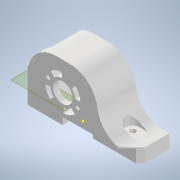
# Autodesk Inventor part: Intake90tdriev
Saved by Autodesk Inventor 2020 (Build 240168000, 168)
## iProperties
Created: 2020-03-03
Part Number: Intake90tdriev
Material: Generic
Document SubType Name: Modeling
Designer: srini
Density: 1 g/cm^3
Appearance: Default
Author: srini
Autodesk Inventor part; units mm, degrees
ref_plane "YZ Plane" through (0, 0, 0) normal (1, 0, 0) x (0, 1, 0)
ref_plane "XZ Plane" through (0, 0, 0) normal (0, 1, 0) x (-1, 0, 0)
ref_plane "XY Plane" through (0, 0, 0) normal (0, 0, 1) x (1, 0, 0)
sketch "Sketch1" plane through (0, 0, 0) normal (0, 0, 1) x (1, 0, 0)
  circle A0 centre (-31.75, -41.275) radius 14.2875 projected
  circle A1 centre (-18.8128, 31.24) radius 8.75 construction
  circle A2 centre (-18.8128, 31.24) radius 8.95
  line L0 (-50.5628, 57.15) -> (12.9372, 57.15)
  line L1 (12.9372, 57.15) -> (12.9372, 0)
  line L2 (12.9372, 0) -> (-50.5628, 0)
  line L3 (-50.5628, 0) -> (-50.5628, 57.15)
  line L4 (450.85, 0) -> (-107.95, 0) projected
  circle A3 centre (-18.8128, 31.24) radius 22.15 construction
  circle A4 centre (-18.8128, 31.24) radius 22.35
  line L5 (-50.5628, 0) -> (-63.5, 0)
  line L6 (-63.5, 0) -> (-63.5, 25.4)
  line L7 (-63.5, 25.4) -> (-50.5628, 25.4)
  line L8 (-50.5628, 25.4) -> (-50.5628, 0)
  line L9 (12.9372, 0) -> (43.4172, 0)
  line L10 (43.4172, 0) -> (43.4172, 12.7)
  line L11 (43.4172, 12.7) -> (12.9372, 12.7)
  line L12 (12.9372, 12.7) -> (12.9372, 0)
  line L13 (-63.5, -1.5266) -> (-63.5, -23.8734) projected
  point P0 (0, 0)
  point P1 (-50.5628, 25.4)
  point P2 (-50.5628, 0)
  point P3 (12.9372, 0)
  point P4 (43.4172, 0)
  point P5 (12.9372, 12.7)
  dimension "d0" = 17.5
  dimension "d1" = 17.9
  dimension "d2" = 73.66
  dimension "d3" = 57.15
  dimension "d4" = 44.3
  dimension "d5" = 44.7
  dimension "d6" = 63.5
  dimension "d7" = 31.75
  dimension "d8" = 25.4
  dimension "d58" = 12.7
  dimension "d59" = 30.48
  dimension "d71" = 31.24
  constraints: 24 end point, 6 parallel, 3 horizontal, 3 perpendicular, 2 centre point, 2 collinear, 1 coincident
  measures "d0" diameter of A1
  measures "d1" diameter of A2
  measures "d2" distance of A0.centre A2.centre
  measures "d3" distance of L2.end L0.start
  measures "d4" diameter of A3
  measures "d5" diameter of A4
  measures "d6" distance of L0.start L0.end
  measures "d7" distance from line of A2.centre L3
  measures "d8" distance of L5.end L6.end
  measures "d58" distance of L9.end L10.end
  measures "d59" distance of L10.end L11.end
  measures "d71" vertical distance of point (0, 0) A4.centre
extrude "Extrusion1" add sketch "Sketch1" against normal blind 25.4 contours L0 L1 L2 L3 | L3 L4 L6 L7 | L11 L10 L4 L1 | A4
sketch "Sketch2" plane through (0, 0, -25.4) normal (0, 0, -1) x (-1, 0, 0)
  circle A0 centre (18.8128, 31.24) radius 8.95 projected
  circle A1 centre (18.8128, 31.24) radius 22.35
  point P0 (0, 0)
  dimension "d12" = 44.7
  constraints: 1 centre point, 1 coincident
  measures "d12" diameter of A1
extrude "Extrusion2" cut sketch "Sketch2" against normal blind 20.32
sketch "Sketch3" plane through (0, 0, -25.4) normal (0, 0, -1) x (-1, 0, 0)
  line L0 (-43.4172, 0) -> (63.5, 0) projected
  circle A0 centre (18.8128, 31.24) radius 22.35 projected
  line L1 (63.5, 0) -> (63.5, 25.4) projected
  line L2 (63.5, 25.4) -> (50.5628, 25.4) projected
  line L3 (50.5628, 25.4) -> (50.5628, 57.15) projected
  line L4 (50.5628, 57.15) -> (-12.9372, 57.15) projected
  line L5 (-12.9372, 57.15) -> (-12.9372, 12.7) projected
  line L6 (-12.9372, 12.7) -> (-43.4172, 12.7) projected
  line L7 (-43.4172, 12.7) -> (-43.4172, 0) projected
  point P0 (0, 0)
ref_plane "Work Plane1" through (-63.5004, -61.913, -35.052) normal (0, 0, -1) x (0, 1, 0)
extrude "Extrusion3" add sketch "Sketch3" along normal up to surface (9.652 mm away)
fillet "Fillet1" radius 25.4 2 edges at (-50.5628, 57.15, -17.526) (12.9372, 57.15, -17.526)
fillet "Fillet2" radius 25.4 2 edges at (-50.5628, 25.4, -17.526) (12.9372, 12.7, -17.526)
chamfer "Chamfer1" distance 12.7 angle 45 2 edges at (-63.5, 12.7, 0) (43.4172, 6.35, 0)
sketch "Sketch4" plane through (-63.5, 25.4, -35.052) normal (0, 1, 0) x (1, 0, 0)
  line L0 (514.35, -2.286) -> (-44.45, -2.286) projected
  line L1 (0, -22.352) -> (0, 0) projected
  line L2 (116.9864, -22.352) -> (116.9864, 0) projected
  circle A0 centre (12.2114, -14.986) radius 2.5781
  circle A1 centre (102.3814, -14.986) radius 2.5781
  line L3 (63.7064, -35.052) -> (45.8064, -35.052) projected
  line L4 (54.7564, -35.052) -> (54.7564, -21.2644)
  point P0 (63.5, -35.052)
  dimension "d26" = 42.545
  dimension "d27" = 47.625
  dimension "d28" = 12.7
  dimension "d29" = 12.7
  dimension "d30" = 5.1562
  constraints: 2 centre point, 2 end point, 1 equal radius, 1 midpoint, 1 vertical
  measures "d26" distance from line of A0.centre L4
  measures "d27" distance from line of A1.centre L4
  measures "d28" distance from line of A0.centre L0
  measures "d29" distance from line of A1.centre L0
  measures "d30" diameter of A0
extrude "Extrusion4" [suppressed]
sketch "Sketch5" plane through (-63.5, 25.4, -35.052) normal (0, 1, 0) x (1, 0, 0)
  circle A0 centre (12.2114, -14.986) radius 2.5781 projected
  circle A1 centre (12.2114, -14.986) radius 6.35
  circle A2 centre (102.3814, -14.986) radius 2.5781 projected
  circle A3 centre (102.3814, -14.986) radius 6.35
  point P0 (63.5, -35.052)
  point P1 (0, -15.9438)
  point P2 (0, -14.0282)
  dimension "d33" = 12.7
  dimension "d34" = 12.7
  constraints: 2 centre point, 2 coincident, 1 other
  measures "d33" diameter of A1
  measures "d34" diameter of A3
extrude "Extrusion5" [suppressed]
sketch "Sketch6" plane through (0, 0, 0) normal (0, 0, 1) x (1, 0, 0)
  line L0 (-17.8812, 15.2671) -> (-18.1549, 19.9592) projected
  arc A0 (-17.8812, 15.2671) -> (-7.832, 19.6029) centre (-18.8128, 31.24) ccw projected
  line L1 (-7.832, 19.6029) -> (-11.0576, 23.0213) projected
  arc A1 (-18.1549, 19.9592) -> (-11.0576, 23.0213) centre (-18.8128, 31.24) ccw projected
  line L2 (-2.84, 32.1716) -> (-7.532, 31.898) projected
  arc A2 (-2.84, 32.1716) -> (-7.1758, 42.2208) centre (-18.8128, 31.24) ccw projected
  line L3 (-7.1758, 42.2208) -> (-10.5941, 38.9952) projected
  arc A3 (-7.532, 31.898) -> (-10.5941, 38.9952) centre (-18.8128, 31.24) ccw projected
  line L4 (-19.4708, 42.5208) -> (-19.7445, 47.2129) projected
  arc A4 (-19.7445, 47.2129) -> (-29.7937, 42.8771) centre (-18.8128, 31.24) ccw projected
  line L5 (-26.568, 39.4587) -> (-29.7937, 42.8771) projected
  arc A5 (-19.4708, 42.5208) -> (-26.568, 39.4587) centre (-18.8128, 31.24) ccw projected
  line L6 (-30.0937, 30.582) -> (-34.7857, 30.3084) projected
  arc A6 (-34.7857, 30.3084) -> (-30.4499, 20.2592) centre (-18.8128, 31.24) ccw projected
  line L7 (-27.0315, 23.4848) -> (-30.4499, 20.2592) projected
  arc A7 (-30.0937, 30.582) -> (-27.0315, 23.4848) centre (-18.8128, 31.24) ccw projected
  circle A8 centre (-32.2888, 36.5924) radius 1.65 projected
  circle A9 centre (-5.3368, 25.8876) radius 1.65 projected
  point P0 (0, 0)
extrude "Extrusion6" cut sketch "Sketch6" against normal through all
sketch "Sketch7" plane through (43.4172, 0, -35.052) normal (0, 0, -1) x (-1, 0, 0)
  line L0 (92.2212, 54.3381) -> (76.8128, 48.2059)
  line L1 (76.8128, 48.2059) -> (84.487, 28.923)
  line L2 (84.487, 28.923) -> (99.8954, 35.0553)
  line L3 (99.8954, 35.0553) -> (92.2212, 54.3381)
  line L4 (86.8955, 49.4848) -> (86.916, 49.5323) projected
  line L5 (86.8955, 49.4848) -> (83.8448, 48.2707) projected
  line L6 (83.8448, 48.2707) -> (83.7035, 48.2517) projected
  line L7 (83.7035, 48.2517) -> (80.1568, 46.8402) projected
  line L8 (80.1542, 46.8413) -> (80.1568, 46.8402) projected
  line L9 (80.1542, 46.8413) -> (86.916, 49.5323) projected
  line L10 (92.7253, 34.9354) -> (92.6777, 34.9559) projected
  line L11 (92.7253, 34.9354) -> (85.9635, 32.2444) projected
  line L12 (85.9635, 32.2444) -> (85.9646, 32.247) projected
  line L13 (85.9646, 32.247) -> (89.5113, 33.6585) projected
  line L14 (89.5113, 33.6585) -> (89.627, 33.7418) projected
  line L15 (89.627, 33.7418) -> (92.6777, 34.9559) projected
  point P0 (43.4172, 0)
  dimension "d39" = 2.54
  dimension "d40" = 2.54
  constraints: 8 end point, 3 parallel, 1 perpendicular
  measures "d39" distance between parallel lines of L0 L5
  measures "d40" distance between parallel lines of L2 L11
extrude "Extrusion7" cut sketch "Sketch7" against normal blind 25.4 contours L3 L2 L1 L0 | L5 L6 L9 L4 | L11 L12 L13 L14 L15 L10
fillet "Fillet3" radius 6.35 2 edges at (-33.4044, 48.1839, -9.652) (-41.059, 28.9504, -9.652)
fillet "Fillet4" radius 2.54 1 edges at (-41.311, 51.356, -22.352)
fillet "Fillet5" radius 2.54 2 edges at (-37.5848, 53.9052, -9.6617) (-44.724, 47.9525, -9.652)
sketch "Sketch8" plane through (5.3668, 0, -35.052) normal (0, 0, -1) x (-1, 0, 0)
  line L0 (68.8668, 0) -> (-38.0504, 0) projected
  line L1 (68.8668, 0) -> (5.3668, 0)
  line L2 (5.3668, 0) -> (5.3668, 5.5562)
  line L3 (5.3668, 5.5562) -> (68.8668, 5.5562)
  line L4 (68.8668, 5.5562) -> (68.8668, 0)
  line L5 (5.3668, 5.5562) -> (24.4168, 5.5562)
  line L6 (24.4168, 5.5562) -> (24.4168, 11.9062)
  line L7 (24.4168, 11.9062) -> (5.3668, 11.9062)
  line L8 (5.3668, 11.9062) -> (5.3668, 5.5562)
  point P0 (5.3668, 0)
  point P1 (24.4168, 5.5562)
  dimension "d75" = 5.5563
  dimension "d76" = 63.5
  dimension "d77" = 19.05
  dimension "d80" = 6.35
  constraints: 16 end point, 4 parallel, 2 horizontal, 2 perpendicular
  measures "d75" distance of L3.end L0.start
  measures "d76" distance of L2.end L3.end
  measures "d77" distance of L6.end L7.end
  measures "d80" distance of L7.end L2.end
extrude "Extrusion8" cut sketch "Sketch8" against normal through all
sketch "Sketch9" plane through (-63.5, 25.4, -35.052) normal (-1, 0, 0) x (0, 0, 1)
  line L0 (8.636, -18.5738) -> (21.336, -18.5738)
  line L1 (21.336, -18.5738) -> (21.336, -22.059)
  line L2 (21.336, -22.059) -> (8.636, -22.059)
  line L3 (8.636, -22.059) -> (8.636, -18.5738)
  line L4 (0, -19.8437) -> (22.352, -19.8438) projected
  arc A0 (21.336, -18.5738) -> (8.636, -18.5738) centre (14.986, -22.7859) ccw
  line L5 (12.4079, -19.8438) -> (17.5641, -19.8438) projected
  point P0 (35.052, -25.4)
  point P1 (12.4079, -12.7)
  point P2 (17.5641, -12.7)
  point P3 (12.4079, 0)
  point P4 (17.5641, 0)
  point P5 (14.986, -0.7938)
  point P6 (12.4079, 0)
  point P7 (17.5641, 0)
  dimension "d49" = 1.27
  dimension "d50" = 12.7
  dimension "d52" = 7.62
  constraints: 8 end point, 2 parallel, 2 point on circle, 1 centre point, 1 horizontal, 1 perpendicular, 1 vertical alignment
  measures "d49" distance between parallel lines of L4 L0
  measures "d50" distance of L1.end L2.end
  measures "d52" radius of A0
extrude "Extrusion9" cut sketch "Sketch9" against normal blind 63.5
sketch "Sketch11" plane through (37.9387, 12.7, -35.052) normal (0, 1, 0) x (1, 0, 0)
  circle A0 centre (-9.1266, -14.986) radius 2.5781 projected
  circle A1 centre (-9.1266, -14.986) radius 6.35
  point P0 (-37.9387, -35.052)
  dimension "d72" = 12.7
  constraints: 1 centre point, 1 coincident
  measures "d72" diameter of A1
extrude "Extrusion11" cut sketch "Sketch11" along normal blind 25.4 contours A0 | A1
sketch "Sketch12" plane through (0, 0, 0) normal (0, 0, 1) x (1, 0, 0)
  line L0 (-7.6, 11.9063) -> (-19.05, 11.9063) projected
  line L1 (0, 11.9063) -> (57.7182, 11.9063)
  line L2 (57.7182, 11.9063) -> (57.7182, -1.1848)
  line L3 (57.7182, -1.1848) -> (0, -1.1848)
  line L4 (0, -1.1848) -> (0, 11.9063)
  point P0 (0, 0)
  constraints: 8 end point, 2 parallel, 1 horizontal, 1 perpendicular
extrude "Extrusion12" cut sketch "Sketch12" against normal blind 8.7313
sketch "Sketch13" plane through (43.4172, 0, -35.052) normal (0, -1, 0) x (1, 0, 0)
  circle A0 centre (-94.615, 14.986) radius 2.54
  circle A1 centre (-18.415, 14.986) radius 2.54
  line L0 (407.4328, 27.686) -> (-151.3672, 27.686) projected
  line L1 (0, 22.352) -> (0, 0) projected
  point P0 (-43.4172, 35.052)
  dimension "d81" = 12.7
  dimension "d82" = 76.2
  dimension "d83" = 18.415
  dimension "d84" = 5.08
  constraints: 2 centre point, 1 equal radius, 1 horizontal alignment
  measures "d81" distance from line of A1.centre L0
  measures "d82" distance of A0.centre A1.centre
  measures "d83" distance from line of A1.centre L1
  measures "d84" diameter of A1
extrude "Extrusion13" cut sketch "Sketch13" against normal through all both and the other way through all
sketch "Sketch14" plane through (28.8122, 12.7, -20.066) normal (0, 1, 0) x (1, 0, 0)
  circle A0 centre (-3.81, 0) radius 2.54 projected
  circle A1 centre (-3.81, 0) radius 6.35
  point P0 (-28.8122, -20.066)
  point P1 (-6.35, 0)
  dimension "d87" = 12.7
  constraints: 1 centre point, 1 coincident, 1 horizontal alignment
  measures "d87" diameter of A1
extrude "Extrusion14" cut sketch "Sketch14" along normal blind 25.4 contours A0 | A1
ref_plane "Work Plane2" through (-50.8, 18.2563, 0) normal (0, -1, 0) x (1, 0, 0)
sketch "Sketch15" plane through (-50.8, 18.2563, 0) normal (0, -1, 0) x (1, 0, 0)
  point P0 (50.8, 0)
sketch "Sketch16" plane through (-50.8, 18.2563, 0) normal (0, -1, 0) x (1, 0, 0)
  arc A0 (-1.9555, -22.0723) -> (-1.9555, -18.0597) centre (-0.3978, -20.066) ccw projected
  circle A1 centre (-0.3978, -20.066) radius 6.35
  point P0 (50.8, 0)
  dimension "d91" = 12.7
  constraints: 1 centre point, 1 coincident
  measures "d91" diameter of A1
extrude "Extrusion15" cut sketch "Sketch16" against normal through all
fillet "Fillet6" radius 3.175 2 edges at (-52.7555, 33.5737, -30.637) (-52.7555, 33.5737, -10.511)
chamfer "Chamfer6" distance 1.27 angle 45 2 edges at (-41.275, 5.5563, -13.716) (-41.275, 5.5563, -26.416)
sketch "Sketch17" plane through (43.4172, 0, -35.052) normal (0, -1, 0) x (1, 0, 0)
  line L0 (-72.0152, 14.986) -> (-61.2389, 25.7623)
  line L1 (-61.2389, 25.7623) -> (-50.4626, 14.986)
  line L2 (-50.4626, 14.986) -> (-61.2389, 4.2097)
  line L3 (-61.2389, 4.2097) -> (-72.0152, 14.986)
  line L4 (-94.2172, 35.052) -> (-62.4672, 35.052) projected
  circle A0 centre (-18.415, 14.986) radius 2.54 projected
  point P0 (-43.4172, 35.052)
  dimension "d98" = 45
  dimension "d99" = 15.24
  constraints: 8 end point, 2 parallel, 2 perpendicular, 1 horizontal alignment
  measures "d98" angle of L0 L4
  measures "d99" distance of L2.end L0.start
extrude "Extrusion16" cut sketch "Sketch17" against normal blind 25.4 contours L0 L1 L2 L3
fillet "Fillet7" radius 3.175 1 edges at (-28.598, 10.69, -20.066)
fillet "Fillet8" radius 1.27 2 edges at (-7.6, 11.9063, -27.8363) (-7.6, 11.9063, -12.2957)
equation "\"d7\" = 0.5 * d6"
equation "\"d12\" = d5"
equation "\"d40\" = d39"
body "Solid1"
